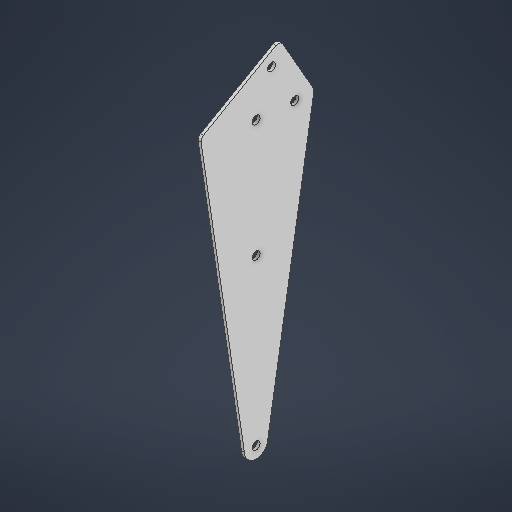
# Autodesk Inventor part: prerollernew
Saved by Autodesk Inventor 2025.2 (Build 292293000, 293)
## iProperties
Created: 2025-04-06
Part Number: prerollernew
Material: Generic
Document SubType Name: Modeling
Designer: roejo
Density: 1 g/cm^3
Appearance: Default
Author: roejo
Autodesk Inventor part; units mm, degrees
ref_plane "YZ Plane" through (0, 0, 0) normal (1, 0, 0) x (0, 1, 0)
ref_plane "XZ Plane" through (0, 0, 0) normal (0, 1, 0) x (-1, 0, 0)
ref_plane "XY Plane" through (0, 0, 0) normal (0, 0, 1) x (1, 0, 0)
sketch "Sketch1" plane through (0, 0, 0) normal (1, 0, 0) x (0, 1, 0)
  circle A0 centre (-86.8757, 0.9387) radius 2.1844
  circle A1 centre (2.0243, 0.9387) radius 2.1844
  circle A2 centre (65.5243, 0.9387) radius 2.1844
  circle A3 centre (64.1826, -19.9575) radius 2.1844
  circle A4 centre (86.2299, -7.3449) radius 2.1844
  line L0 (65.9484, -29.438) -> (95.1218, -12.7487)
  circle A5 centre (64.1826, -19.9575) radius 2.1844
  circle A6 centre (65.5243, 0.9387) radius 2.1844
  circle A7 centre (86.2299, -7.3449) radius 2.1844
  circle A8 centre (2.0243, 0.9387) radius 2.1844
  circle A9 centre (-86.8757, 0.9387) radius 2.1844
  circle A10 centre (-86.8757, 0.9387) radius 6.35
  line L1 (-86.8757, -5.4113) -> (63.0678, -30.2634)
  line L2 (65.1635, -29.887) -> (94.0863, -13.341)
  line L3 (95.0298, -9.8751) -> (72.5412, 29.4356)
  line L4 (69.9617, 30.6865) -> (-86.8757, 7.2887)
  arc A11 (63.0678, -30.2634) -> (65.1635, -29.887) centre (63.5869, -27.1311) ccw
  arc A12 (94.0863, -13.341) -> (95.0298, -9.8751) centre (92.8251, -11.1363) ccw
  arc A13 (72.5412, 29.4356) -> (69.9617, 30.6865) centre (70.3364, 28.1743) ccw
  point P0 (0, 0)
  point P1 (96.291, -12.0798)
  dimension "d0" = 12.7
  dimension "d1" = 3.175
  dimension "d2" = 2.54
  constraints: 14 centre point, 10 end point, 8 point on circle, 6 coincident, 6 equal radius, 6 tangent, 3 point on line, 1 perpendicular
  measures "d0" diameter of A10
  measures "d1" radius of A11
  measures "d2" radius of A12
extrude "Extrusion1" add sketch "Sketch1" along normal blind 1.5875
body "Solid1"
